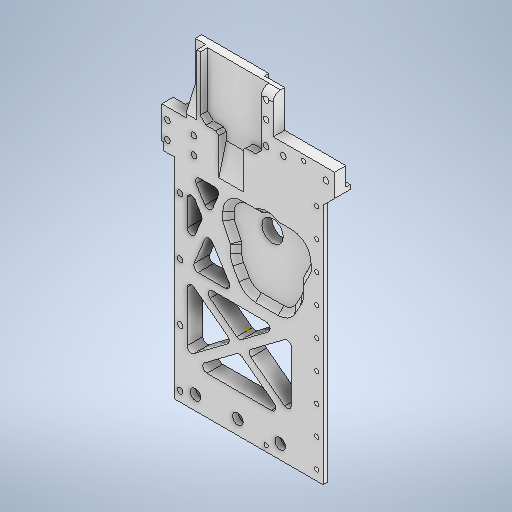
# Autodesk Inventor part: BottomSideMountRight
Saved by Autodesk Inventor 2026.2 (Build 302298000, 298)
## iProperties
Created: 2026-03-09
Part Number: BottomSideMountRight
Material: ABS Plastic
Document SubType Name: Modeling
Designer: gaoet
Density: 1.06 g/cm^3
Appearance: Smooth - White
Author: gaoet
Autodesk Inventor part; units mm, degrees
(part 1 of 2)
ref_plane "YZ Plane" through (0, 0, 0) normal (1, 0, 0) x (0, 1, 0)
ref_plane "XZ Plane" through (0, 0, 0) normal (0, 1, 0) x (-1, 0, 0)
ref_plane "XY Plane" through (0, 0, 0) normal (0, 0, 1) x (1, 0, 0)
sketch "Sketch1" plane through (0, 0, 0) normal (0, 0, 1) x (1, 0, 0)
  line L0 (56.625, -110) -> (-56.625, -110)
  line L1 (-56.625, -110) -> (-56.625, 110)
  line L2 (-56.625, 110) -> (56.625, 110)
  line L3 (56.625, 110) -> (56.625, -110)
  line L4 (56.625, -110) -> (-56.625, 110) construction
  line L5 (-56.625, -110) -> (56.625, 110) construction
  line L6 (-56.625, 110) -> (-47.875, 110)
  line L7 (-47.875, 110) -> (-47.875, 82)
  line L8 (-47.875, 82) -> (-56.625, 82)
  line L9 (-56.625, 82) -> (-56.625, 110)
  line L10 (-47.875, 82) -> (-47.875, -110)
  point P0 (0, 0)
  point P1 (-56.625, 82)
  dimension "d0" = 113.25
  dimension "d1" = 220
  dimension "d4" = 8.75
  dimension "d5" = 28
  constraints: 22 end point, 4 parallel, 2 horizontal, 2 midpoint, 2 perpendicular, 1 point on line, 1 vertical
  measures "d0" distance of L1.end L2.end
  measures "d1" distance of L0.end L1.end
  measures "d4" distance of L7.end L8.end
  measures "d5" distance of L6.end L7.end
extrude "Extrusion1" add sketch "Sketch1" along normal blind 8 contours L0 L10 L7 L2 L3 | L8 L1 L2 L7
sketch "Sketch2" plane through (0, 0, 8) normal (0, 0, 1) x (1, 0, 0)
  line L0 (-52.625, 102) -> (-34.125, 102)
  line L1 (-34.125, 102) -> (-34.125, 90)
  line L2 (-34.125, 90) -> (-52.625, 90)
  line L3 (-52.625, 90) -> (-52.625, 102)
  line L4 (-56.625, 110) -> (-56.625, 82) projected
  line L5 (56.625, 110) -> (-56.625, 110) projected
  point P0 (0, 0)
  dimension "d6" = 12
  dimension "d7" = 18.5
  dimension "d8" = 4
  dimension "d9" = 8
  constraints: 8 end point, 2 parallel, 1 horizontal, 1 perpendicular
  measures "d6" distance of L0.end L1.end
  measures "d7" distance of L0.start L0.end
  measures "d8" distance between parallel lines of L4 L3
  measures "d9" distance between parallel lines of L5 L0
hole "Hole1" at (-34.125, 102, 8) at (-34.125, 90, 8) at (-52.625, 90, 8) at (-52.625, 102, 8) direction (0, 0, -1) diameter 4 end through all
sketch "Sketch3" plane through (0, 0, 8) normal (0, 0, 1) x (1, 0, 0)
  circle A0 centre (-52.625, 102) radius 2 projected
  circle A1 centre (-52.625, 90) radius 2 projected
  circle A2 centre (-34.125, 90) radius 2 projected
  circle A3 centre (-34.125, 102) radius 2 projected
  line L0 (56.625, 110) -> (-56.625, 110) projected
  line L1 (-56.625, 110) -> (-56.625, 82) projected
  line L2 (-56.625, 82) -> (-47.875, 82) projected
  line L3 (-47.875, 82) -> (-47.875, -110) projected
  line L4 (-47.875, -110) -> (56.625, -110) projected
  line L5 (56.625, -110) -> (56.625, 110) projected
  line L6 (-56.625, 87.5) -> (-55.375, 87.5)
  line L7 (-55.375, 87.5) -> (-55.375, 82)
  point P0 (0, 0)
  dimension "d17" = 1.25
  dimension "d18" = 5.5
  constraints: 4 end point, 2 point on line, 1 horizontal, 1 perpendicular
  measures "d17" distance of L6.start L6.end
  measures "d18" distance of L6.end L7.end
extrude "Extrusion2" cut sketch "Sketch3" against normal blind 8 contours L6 L7 L2 L1
sketch "Sketch4" plane through (-47.875, -110, 0) normal (0, -1, 0) x (1, 0, 0)
  line L0 (0, 0) -> (104.5, 0) projected
  line L1 (104.5, 0) -> (104.5, 8) projected
  line L2 (0, 8) -> (104.5, 8) projected
  line L3 (0, 0) -> (0, 8) projected
  line L4 (104.5, 0) -> (89.25, 0)
  line L5 (89.25, 0) -> (89.25, 5)
  line L6 (89.25, 5) -> (104.5, 5)
  line L7 (104.5, 5) -> (104.5, 0)
  line L8 (89.25, 3.5) -> (95.5, 3.5)
  line L9 (95.5, 3.5) -> (95.5, 5)
  point P0 (47.875, 0)
  point P1 (89.25, 0)
  dimension "d21" = 15.25
  dimension "d22" = 5
  dimension "d25" = 1.5
  dimension "d26" = 9
  constraints: 12 end point, 2 horizontal, 2 parallel, 2 perpendicular, 2 point on line
  measures "d21" distance of L5.end L6.end
  measures "d22" distance of L4.end L5.end
  measures "d25" distance of L8.end L9.end
  measures "d26" distance between parallel lines of L1 L9
extrude "Extrusion3" cut sketch "Sketch4" against normal through all contours L5 L8 L9 L6 L1 L0
chamfer "Chamfer2" distance 5 angle 45 1 edges at (-51.625, 82, 0)
sketch "Sketch5" plane through (0, 0, 8) normal (0, 0, 1) x (1, 0, 0)
  line L0 (-56.625, 87.5) -> (-55.375, 87.5) projected
  line L1 (-55.375, 87.5) -> (-55.375, 82) projected
  line L2 (-55.375, 82) -> (-47.875, 82) projected
  line L3 (-47.875, 82) -> (-47.875, -110) projected
  line L4 (-47.875, -110) -> (56.625, -110) projected
  line L5 (56.625, -110) -> (56.625, 110) projected
  line L6 (56.625, 110) -> (-56.625, 110) projected
  line L7 (-56.625, 110) -> (-56.625, 87.5) projected
  circle A0 centre (-34.125, 102) radius 2 projected
  circle A1 centre (-34.125, 90) radius 2 projected
  circle A2 centre (-52.625, 90) radius 2 projected
  circle A3 centre (-52.625, 102) radius 2 projected
  line L8 (56.625, -65) -> (-47.875, -65)
  point P0 (0, 0)
  dimension "d33" = 45
  constraints: 2 end point, 2 point on line, 1 perpendicular
  measures "d33" distance between parallel lines of L8 L4
extrude "Extrusion4" cut sketch "Sketch5" against normal blind 25.4 contours L5 L4 L3 L8
sketch "Sketch6" plane through (-56.625, 110, 8) normal (0, 1, 0) x (1, 0, 0)
  line L0 (98, 4.5) -> (98, 8) projected
  line L1 (98, 8) -> (0, 8) projected
  line L2 (0, 8) -> (0, 0) projected
  line L3 (113.25, 0) -> (0, 0) projected
  line L4 (113.25, 3) -> (113.25, 0) projected
  line L5 (113.25, 3) -> (104.25, 3) projected
  line L6 (104.25, 3) -> (104.25, 4.5) projected
  line L7 (104.25, 4.5) -> (98, 4.5) projected
  line L8 (17, 0) -> (17, 8)
  line L9 (113.25, 3) -> (113.25, 8)
  line L10 (113.25, 8) -> (98, 8)
  point P0 (56.625, 8)
  point P1 (113.25, 1.5)
  dimension "d36" = 96.25
  constraints: 6 end point, 2 point on line, 1 horizontal, 1 midpoint, 1 perpendicular, 1 vertical
  measures "d36" distance from line of point (113.25, 1.5) L8
extrude "Extrusion5" add sketch "Sketch6" along normal blind 45 contours L7 L6 L5 L4 L3 L8 L1 L0 | L0 L10 L9 L5 L6 L7
sketch "Sketch7" plane through (0, 0, 8) normal (0, 0, 1) x (1, 0, 0)
  circle A0 centre (-52.625, 102) radius 2 projected
  circle A1 centre (-52.625, 90) radius 2 projected
  circle A2 centre (-34.125, 90) radius 2 projected
  circle A3 centre (-34.125, 102) radius 2 projected
  line L0 (-47.875, -65) -> (56.625, -65) projected
  line L1 (56.625, -65) -> (56.625, 155) projected
  line L2 (-39.625, 155) -> (56.625, 155) projected
  line L3 (-39.625, 110) -> (-39.625, 155) projected
  line L4 (-39.625, 110) -> (-56.625, 110) projected
  line L5 (-56.625, 110) -> (-56.625, 87.5) projected
  line L6 (-56.625, 87.5) -> (-55.375, 87.5) projected
  line L7 (-55.375, 87.5) -> (-55.375, 82) projected
  line L8 (-55.375, 82) -> (-47.875, 82) projected
  line L9 (-47.875, 82) -> (-47.875, -65) projected
  line L10 (56.625, 129) -> (21.625, 129)
  line L11 (21.625, 129) -> (21.625, 155)
  point P0 (0, 0)
  dimension "d39" = 26
  dimension "d40" = 35
  constraints: 4 end point, 2 point on line, 1 horizontal, 1 perpendicular
  measures "d39" distance of L10.end L11.end
  measures "d40" distance of L10.start L10.end
extrude "Extrusion6" cut sketch "Sketch7" against normal blind 25.4 contours L10 L11 L2 L1
sketch "Sketch8" plane through (0, 0, 8) normal (0, 0, 1) x (1, 0, 0)
  line L0 (56.625, 129) -> (21.625, 129) projected
  line L1 (21.625, 129) -> (21.625, 155) projected
  line L2 (56.625, -65) -> (56.625, 129) projected
  line L3 (-39.625, 155) -> (21.625, 155) projected
  point P0 (0, 0)
  point P1 (28.625, 121)
  point P2 (16.625, 121)
  point P3 (16.625, 137)
  point P4 (16.625, 149)
  point P5 (50.625, 121)
  point P6 (50.625, 121)
  dimension "d46" = 8
  dimension "d47" = 5
  dimension "d49" = 6
  dimension "d50" = 12
  dimension "d51" = 12
  dimension "d59" = 0
  dimension "d60" = 16
  dimension "d94" = 34
  constraints: 2 horizontal alignment, 2 vertical alignment, 1 coincident
  measures "d46" distance from line of L0 point (16.625, 121)
  measures "d47" distance from line of L1 point (16.625, 137)
  measures "d49" distance from line of L3 point (16.625, 149)
  measures "d50" distance of point (16.625, 149) point (16.625, 137)
  measures "d51" distance of point (28.625, 121) point (16.625, 121)
  measures "d59" horizontal distance of point (16.625, 137) point (16.625, 121)
  measures "d60" distance of point (16.625, 137) point (16.625, 121)
  measures "d94" distance of point (16.625, 121) point (50.625, 121)
hole "Hole2" at (28.625, 121, 8) at (16.625, 121, 8) at (16.625, 137, 8) at (16.625, 149, 8) direction (0, 0, -1) diameter 4 end through all
sketch "Sketch11" plane through (56.625, 110, 5) normal (1, 0, 0) x (0, 0, -1)
  line L0 (5, 19) -> (-3, 19) projected
  line L1 (-3, -175) -> (-3, 19) projected
  line L2 (-3, -175) -> (0, -175) projected
  line L3 (0, -175) -> (0, 0) projected
  line L4 (0, 0) -> (5, 0) projected
  line L5 (5, 0) -> (5, 19) projected
  line L6 (0, -175) -> (0, 0) projected
  line L7 (0, -30) -> (5, -30)
  line L8 (1.5, -175) -> (5, -175) projected
  line L9 (5, 0) -> (5, -175) projected
  line L10 (1.5, 0) -> (5, 0) projected
  line L11 (1.5, -175) -> (1.5, 0) projected
  point P0 (5, -110)
  point P1 (0, -30)
  dimension "d71" = 30
  constraints: 2 end point, 1 horizontal, 1 point on line
  measures "d71" distance between parallel lines of L4 L7
extrude "Extrusion9" add sketch "Sketch11" against normal up to surface (15.25 mm away) contours L9 L7 L11 L4 | L11 L7 L3 L4
sketch "Sketch13" plane through (-47.875, -65, 8) normal (0, -1, 0) x (1, 0, 0)
  line L0 (89.25, -8) -> (0, -8) projected
  line L1 (89.25, -4.5) -> (89.25, -8) projected
  line L2 (95.5, -4.5) -> (89.25, -4.5) projected
  line L3 (95.5, -3) -> (95.5, -4.5) projected
  line L4 (104.5, -3) -> (95.5, -3) projected
  line L5 (104.5, 0) -> (104.5, -3) projected
  line L6 (0, 0) -> (104.5, 0) projected
  line L7 (0, -8) -> (0, 0) projected
  line L8 (95.5, -4.5) -> (95.5, -7.5)
  line L9 (95.5, -7.5) -> (104.5, -7.5)
  line L10 (95.5, -7.5) -> (95.5, -8)
  line L11 (95.5, -4.5) -> (95.5, -3) projected
  line L12 (89.25, -4.5) -> (95.5, -4.5) projected
  line L13 (89.25, -8) -> (89.25, -4.5) projected
  line L14 (104.5, -8) -> (89.25, -8) projected
  line L15 (104.5, -3) -> (104.5, -8) projected
  line L16 (95.5, -3) -> (104.5, -3) projected
  point P0 (47.875, -8)
  dimension "d77" = 4.5
  constraints: 6 end point, 2 perpendicular, 2 point on line, 2 vertical
  measures "d77" distance between parallel lines of L4 L9
extrude "Extrusion11" [suppressed]
sketch "Sketch14" plane through (0, 0, 0) normal (0, 0, -1) x (-1, 0, 0)
  line L0 (-56.625, 80) -> (-56.625, 129) projected
  line L1 (-21.625, 129) -> (-56.625, 129) projected
  point P0 (0, 0)
  point P1 (-53.125, 125)
  point P2 (-42.875, 125)
  dimension "d81" = 3.5
  dimension "d82" = 4
  dimension "d83" = 10.25
  constraints: 1 horizontal alignment
  measures "d81" distance from line of L0 point (-53.125, 125)
  measures "d82" distance from line of L1 point (-53.125, 125)
  measures "d83" distance of point (-42.875, 125) point (-53.125, 125)
hole "Hole3" at (42.875, 125, 0) direction (0, 0, 1) diameter 3 end through all
sketch "Sketch15" plane through (0, 0, 0) normal (0, 0, -1) x (-1, 0, 0)
  circle A0 centre (-42.875, 125) radius 1.5 projected
  circle A1 centre (-16.625, 149) radius 2 projected
  circle A2 centre (-16.625, 137) radius 2 projected
  circle A3 centre (-16.625, 121) radius 2 projected
  circle A4 centre (-28.625, 121) radius 2 projected
  line L0 (-21.625, 155) -> (-21.625, 129) projected
  line L1 (-21.625, 129) -> (-56.625, 129) projected
  line L2 (-56.625, 80) -> (-56.625, 129) projected
  line L3 (-56.625, 80) -> (-41.375, 80) projected
  line L4 (-41.375, -65) -> (47.875, -65) projected
  line L5 (47.875, 87) -> (47.875, -65) projected
  line L6 (55.375, 87) -> (47.875, 87) projected
  line L7 (55.375, 87) -> (55.375, 87.5) projected
  line L8 (55.375, 87.5) -> (56.625, 87.5) projected
  line L9 (56.625, 110) -> (56.625, 87.5) projected
  line L10 (39.625, 110) -> (56.625, 110) projected
  line L11 (39.625, 110) -> (39.625, 155) projected
  line L12 (-21.625, 155) -> (39.625, 155) projected
  circle A5 centre (52.625, 102) radius 2 projected
  circle A6 centre (52.625, 90) radius 2 projected
  circle A7 centre (34.125, 90) radius 2 projected
  circle A8 centre (34.125, 102) radius 2 projected
  line L13 (-51.5517, 125.725) -> (-49.9784, 123)
  line L14 (-49.9784, 123) -> (-51.5517, 120.275)
  line L15 (-51.5517, 120.275) -> (-54.6983, 120.275)
  line L16 (-54.6983, 120.275) -> (-56.2716, 123)
  line L17 (-56.2716, 123) -> (-54.6983, 125.725)
  line L18 (-54.6983, 125.725) -> (-51.5517, 125.725)
  line L19 (-41.3017, 127.725) -> (-39.7284, 125)
  line L20 (-39.7284, 125) -> (-41.3017, 122.275)
  line L21 (-41.3017, 122.275) -> (-44.4483, 122.275)
  line L22 (-44.4483, 122.275) -> (-46.0216, 125)
  line L23 (-46.0216, 125) -> (-44.4483, 127.725)
  line L24 (-44.4483, 127.725) -> (-41.3017, 127.725)
  line L25 (-41.375, 80) -> (-41.375, -65) projected
  point P0 (0, 0)
  point P1 (-53.125, 123)
  dimension "d91" = 5.45
  constraints: 24 end point, 2 horizontal, 1 coincident, 1 equal length, 26 other
  measures "d91" distance between parallel lines of L15 L18
extrude "Extrusion12" cut sketch "Sketch15" against normal blind 2.5 contours A0 | L19 L20 L21 L22 L23 L24
sketch "Sketch16" plane through (0, 0, 8) normal (0, 0, 1) x (1, 0, 0)
  circle A0 centre (42.875, 125) radius 1.5 projected
  circle A1 centre (16.625, 149) radius 2 projected
  circle A2 centre (16.625, 137) radius 2 projected
  circle A3 centre (16.625, 121) radius 2 projected
  circle A4 centre (28.625, 121) radius 2 projected
  line L0 (56.625, 129) -> (21.625, 129) projected
  line L1 (21.625, 129) -> (21.625, 155) projected
  line L2 (-39.625, 155) -> (21.625, 155) projected
  line L3 (-39.625, 110) -> (-39.625, 155) projected
  line L4 (-39.625, 110) -> (-56.625, 110) projected
  line L5 (-56.625, 110) -> (-56.625, 87.5) projected
  line L6 (-56.625, 87.5) -> (-55.375, 87.5) projected
  line L7 (-55.375, 87.5) -> (-55.375, 82) projected
  line L8 (-55.375, 82) -> (-47.875, 82) projected
  line L9 (-47.875, 82) -> (-47.875, -65) projected
  line L10 (-47.875, -65) -> (56.625, -65) projected
  line L11 (56.625, -65) -> (56.625, 129) projected
  circle A5 centre (-34.125, 102) radius 2 projected
  circle A6 centre (-34.125, 90) radius 2 projected
  circle A7 centre (-52.625, 90) radius 2 projected
  circle A8 centre (-52.625, 102) radius 2 projected
  line L12 (56.625, 129) -> (64.625, 129)
  line L13 (64.625, 129) -> (64.625, 113)
  line L14 (64.625, 113) -> (56.625, 113)
  circle A9 centre (58.625, 121) radius 2
  point P0 (0, 0)
  point P1 (56.625, 121)
  dimension "d98" = 8
  dimension "d104" = 8
  dimension "d105" = 8
  dimension "d106" = 2
  constraints: 6 end point, 2 perpendicular, 1 centre point, 1 coincident, 1 equal radius, 1 horizontal, 1 point on line
  measures "d98" distance of L0.start L12.end
  measures "d104" distance from line of L0 A9.centre
  measures "d105" distance from line of A9.centre L14
  measures "d106" distance from line of L11 A9.centre
extrude "Extrusion13" add sketch "Sketch16" against normal up to surface (8 mm away) contours L12 L13 L14 L11
chamfer "Chamfer4" distance 8 angle 45 1 edges at (56.625, 113, 4)
sketch "Sketch17" plane through (56.625, 80, 0) normal (0, -1, 0) x (1, 0, 0)
  line L0 (-9, 3.5) -> (-9, 5) projected
  line L1 (-15.25, 3.5) -> (-9, 3.5) projected
  line L2 (-15.25, 0) -> (-15.25, 3.5) projected
  line L3 (0, 0) -> (-15.25, 0) projected
  line L4 (0, 5) -> (0, 0) projected
  line L5 (-9, 5) -> (0, 5) projected
  point P0 (-56.625, 0)
extrude "Extrusion14" cut sketch "Sketch17" against normal blind 27
sketch "Sketch18" plane through (0, 0, 8) normal (0, 0, 1) x (1, 0, 0)
  circle A0 centre (17.125, 67.6) radius 7.5
  line L0 (56.625, -65) -> (56.625, 105) projected
  line L1 (-39.625, 155) -> (21.625, 155) projected
  line L2 (-7.375, 72.6) -> (41.625, 72.6)
  line L3 (41.625, 72.6) -> (41.625, 28.6)
  line L4 (41.625, 28.6) -> (-7.375, 28.6)
  line L5 (-7.375, 28.6) -> (-7.375, 72.6)
  line L6 (-7.375, 61.6) -> (8.125, 28.6)
  line L7 (41.625, 61.6) -> (26.125, 28.6)
  line L8 (-1.9735, 50.1) -> (36.2235, 50.1)
  line L9 (-1.9735, 50.1) -> (-1.9735, 41.1)
  line L10 (-1.9735, 41.1) -> (5.125, 28.6)
  line L11 (36.2235, 50.1) -> (36.2235, 41.1)
  line L12 (36.2235, 41.1) -> (29.125, 28.6)
  point P0 (0, 0)
  point P1 (-9, 155)
  dimension "d109" = 39.5
  dimension "d110" = 87.4
  dimension "d111" = 15
  dimension "d112" = 49
  dimension "d113" = 39
  dimension "d114" = 24.5
  dimension "d115" = 11
  dimension "d116" = 18
  dimension "d119" = 5
  dimension "d120" = 17.5
  dimension "d121" = 9
  dimension "d122" = 24
  constraints: 22 end point, 8 point on line, 2 equal length, 2 horizontal, 2 horizontal alignment, 2 parallel, 2 vertical, 1 centre point, 1 midpoint, 1 perpendicular
  measures "d109" distance from line of A0.centre L0
  measures "d110" vertical distance of point (-9, 155) A0.centre
  measures "d111" diameter of A0
  measures "d112" distance of L3.end L4.end
  measures "d113" distance from line of L4 A0.centre
  measures "d114" distance from line of L3 A0.centre
  measures "d115" distance of L2.start L6.start
  measures "d116" distance of L7.end L6.end
  measures "d119" distance from line of A0.centre L2
  measures "d120" distance from line of A0.centre L8
  measures "d121" distance of L8.start L9.end
  measures "d122" distance of L12.end L10.end
extrude "Extrusion15" cut sketch "Sketch18" against normal blind 4 contours A0 L2 | A0 L2 L3 L7 L8 L6 L5 | L11 L12 L4 L7 | L7 L4 L6 L8 | L6 L4 L10 L9 picked at (19.5586, 67.0082)
fillet "Fillet1" radius 7 2 edges at (41.625, 72.6, 6) (-7.375, 72.6, 6)
extrude "Extrusion16" cut sketch "Sketch18" against normal blind 17.5 contours A0 L2 | L2 A0
fillet "Fillet2" radius 7 8 edges at (-1.9735, 50.1, 6) (-1.9735, 41.1, 6) (36.2235, 50.1, 6) (36.2235, 41.1, 6) (5.125, 28.6, 6) (29.125, 28.6, 6) (11.5348, 72.6, 6) (22.7152, 72.6, 6)
sketch "Sketch20" plane through (0, 0, 0) normal (0, 0, -1) x (-1, 0, 0)
  line L0 (47.875, 87) -> (47.875, -65) projected
  line L1 (-41.375, -65) -> (47.875, -65) projected
  point P0 (0, 0)
  point P1 (43.75, 62)
  point P2 (43.75, 22)
  point P3 (43.75, -18)
  point P4 (43.75, -58)
  dimension "d129" = 40
  dimension "d130" = 40
  dimension "d131" = 40
  dimension "d132" = 4.125
  dimension "d133" = 7
  constraints: 3 vertical alignment
  measures "d129" distance of point (43.75, 22) point (43.75, 62)
  measures "d130" distance of point (43.75, 22) point (43.75, -18)
  measures "d131" distance of point (43.75, -58) point (43.75, -18)
  measures "d132" distance from line of L0 point (43.75, 22)
  measures "d133" distance from line of L1 point (43.75, -58)
hole "Hole4" at (-43.75, 62, 0) at (-43.75, 22, 0) at (-43.75, -18, 0) at (-43.75, -58, 0) direction (0, 0, 1) diameter 4 depth 12
sketch "Sketch21" plane through (56.625, -65, 5) normal (0, 0, -1) x (-1, 0, 0)
  point P0 (56.625, 65)
sketch "Sketch22" plane through (56.625, -65, 5) normal (0, 0, -1) x (-1, 0, 0)
  line L0 (0, 170) -> (0, 172) projected
  line L1 (0, 0) -> (9, 0) projected
  line L2 (9, 0) -> (9, 172) projected
  line L3 (9, 172) -> (0, 172) projected
  line L4 (0, 0) -> (0, 170) projected
  point P0 (56.625, 65)
  point P1 (4.5, 167)
  point P2 (4.5, 147)
  point P3 (4.5, 127)
  point P4 (4.5, 107)
  point P5 (4.5, 87)
  point P6 (4.5, 67)
  point P7 (4.5, 47)
  point P8 (4.5, 27)
  point P9 (4.5, 7)
  point P10 (4.5, -13)
  point P11 (4.5, -33)
  dimension "d141" = 5
  dimension "d142" = 9
  dimension "d143" = 4.5
  dimension "d146" = 20
  constraints: 1 vertical, 10 other
  measures "d141" distance from line of L3 point (4.5, 167)
  measures "d142" distance of L2.end L0.end
  measures "d143" distance from line of point (4.5, 167) L2
  measures "d146" distance of point (4.5, 167) point (4.5, 147)
hole "Hole5" at (52.125, -98, 5) at (52.125, -58, 5) at (52.125, -38, 5) at (52.125, -18, 5) at (52.125, 2, 5) at (52.125, 22, 5) at (52.125, 42, 5) at (52.125, 62, 5) at (52.125, 82, 5) at (52.125, 102, 5) direction (0, 0, 1) diameter 3 depth 12
sketch "Sketch23" plane through (0, 0, 0) normal (0, 0, -1) x (-1, 0, 0)
  circle A0 centre (43.75, -58) radius 2 projected
  circle A1 centre (43.75, -18) radius 2 projected
  circle A2 centre (43.75, 22) radius 2 projected
  circle A3 centre (43.75, 62) radius 2 projected
  circle A4 centre (-17.125, 67.6) radius 7.5 projected
  circle A5 centre (34.125, 102) radius 2 projected
  circle A6 centre (34.125, 90) radius 2 projected
  circle A7 centre (52.625, 90) radius 2 projected
  circle A8 centre (52.625, 102) radius 2 projected
  circle A9 centre (-58.625, 121) radius 2 projected
  circle A10 centre (-28.625, 121) radius 2 projected
  circle A11 centre (-16.625, 121) radius 2 projected
  circle A12 centre (-16.625, 137) radius 2 projected
  circle A13 centre (-16.625, 149) radius 2 projected
  line L0 (-44.4483, 122.275) -> (-46.0216, 125) projected
  line L1 (-46.0216, 125) -> (-44.4483, 127.725) projected
  line L2 (-44.4483, 127.725) -> (-41.3017, 127.725) projected
  line L3 (-41.3017, 127.725) -> (-39.7284, 125) projected
  line L4 (-39.7284, 125) -> (-41.3017, 122.275) projected
  line L5 (-41.3017, 122.275) -> (-44.4483, 122.275) projected
  line L6 (-56.625, 105) -> (-56.625, 107) projected
  line L7 (-56.625, 107) -> (-41.375, 107) projected
  line L8 (-41.375, 107) -> (-41.375, -65) projected
  line L9 (-41.375, -65) -> (47.875, -65) projected
  line L10 (47.875, 87) -> (47.875, -65) projected
  line L11 (55.375, 87) -> (47.875, 87) projected
  line L12 (55.375, 87) -> (55.375, 87.5) projected
  line L13 (55.375, 87.5) -> (56.625, 87.5) projected
  line L14 (56.625, 110) -> (56.625, 87.5) projected
  line L15 (39.625, 110) -> (56.625, 110) projected
  line L16 (39.625, 110) -> (39.625, 155) projected
  line L17 (-21.625, 155) -> (39.625, 155) projected
  line L18 (-21.625, 155) -> (-21.625, 129) projected
  line L19 (-21.625, 129) -> (-64.625, 129) projected
  line L20 (-64.625, 129) -> (-64.625, 113) projected
  line L21 (-56.625, 105) -> (-64.625, 113) projected
  line L22 (-64.625, 155) -> (-7.625, 155)
  line L23 (-7.625, 155) -> (-7.625, 116)
  line L24 (-7.625, 116) -> (-64.625, 116)
  line L25 (-64.625, 116) -> (-64.625, 155)
  line L26 (-21.625, 155) -> (39.625, 155) projected
  line L27 (47.875, 87) -> (47.875, 110)
  point P0 (0, 0)
  point P1 (-7.625, 155)
  dimension "d158" = 39
  dimension "d159" = 14
  constraints: 10 end point, 2 parallel, 1 collinear, 1 horizontal, 1 perpendicular, 1 point on line, 1 vertical, 1 vertical alignment
  measures "d158" distance of L22.end L23.end
  measures "d159" distance between parallel lines of L18 L23
extrude "Extrusion18" add sketch "Sketch23" along normal blind 3 contours L21 L20 L24 L23 L17 L16 L15 L27 L10 L9 L8 L7 L6
sketch "Sketch24" plane through (0, 0, -3) normal (0, 0, -1) x (-1, 0, 0)
  line L0 (-56.625, 105) -> (-56.625, 107) projected
  line L1 (-56.625, 107) -> (-41.375, 107) projected
  line L2 (-41.375, 107) -> (-41.375, -65) projected
  line L3 (-41.375, -65) -> (47.875, -65) projected
  line L4 (47.875, -65) -> (47.875, 110) projected
  line L5 (47.875, 110) -> (39.625, 110) projected
  line L6 (39.625, 110) -> (39.625, 155) projected
  line L7 (39.625, 155) -> (-7.625, 155) projected
  line L8 (-7.625, 155) -> (-7.625, 116) projected
  line L9 (-7.625, 116) -> (-64.625, 116) projected
  line L10 (-64.625, 116) -> (-64.625, 113) projected
  line L11 (-64.625, 113) -> (-56.625, 105) projected
  circle A0 centre (34.125, 90) radius 2 projected
  circle A1 centre (34.125, 102) radius 2 projected
  circle A2 centre (-17.125, 67.6) radius 7.5 projected
  circle A3 centre (43.75, 62) radius 2 projected
  circle A4 centre (43.75, 22) radius 2 projected
  circle A5 centre (43.75, -18) radius 2 projected
  circle A6 centre (43.75, -58) radius 2 projected
  line L12 (47.875, -45) -> (-41.375, -45)
  line L13 (39.625, -65) -> (39.625, -45)
  point P0 (0, 0)
  dimension "d162" = 20
  dimension "d177" = 4.125
  dimension "d178" = 4.125
  constraints: 4 end point, 4 point on line, 1 horizontal, 1 vertical
  measures "d162" distance between parallel lines of L3 L12
  measures "d177" distance from line of L4 A6.centre
  measures "d178" distance from line of L13 A6.centre
extrude "Extrusion19" cut sketch "Sketch24" against normal blind 5 contours L12 L13 L3 L2
sketch "Sketch25" plane through (0, 0, 2) normal (0, 0, -1) x (-1, 0, 0)
  line L0 (-41.375, -45) -> (39.625, -45) projected
  line L1 (-41.375, -65) -> (-41.375, -45) projected
  line L2 (39.625, -65) -> (-41.375, -65) projected
  line L3 (39.625, -45) -> (39.625, -65) projected
  point P0 (0, 0)
  point P1 (33, -55)
  point P2 (3.25, -55)
  point P3 (-26.5, -55)
  dimension "d165" = 10
  dimension "d168" = 29.75
  dimension "d169" = 29.75
  constraints: 2 horizontal alignment
  measures "d165" distance from line of L2 point (33, -55)
  measures "d168" distance of point (3.25, -55) point (33, -55)
  measures "d169" distance of point (-26.5, -55) point (3.25, -55)
hole "Hole6" at (-33, -55, 2) at (26.5, -55, 2) at (-3.25, -55, 2) direction (0, 0, 1) diameter 4 depth 30
chamfer "Chamfer5" distance 10 angle 45 1 edges at (-39.625, -45, -0.5)
sketch "Sketch26" plane through (0, 0, 8) normal (0, 0, 1) x (1, 0, 0)
  line L0 (-47.875, -65) -> (56.625, -65) projected
  line L1 (56.625, -65) -> (56.625, 105) projected
  point P0 (0, 0)
  point P1 (16.625, -61)
  dimension "d182" = 4
  dimension "d183" = 40
  measures "d182" distance from line of L0 point (16.625, -61)
  measures "d183" distance from line of L1 point (16.625, -61)
hole "Hole7" at (16.625, -61, 8) direction (0, 0, -1) diameter 3 end through all
sketch "Sketch28" plane through (0, 0, -3) normal (0, 0, -1) x (-1, 0, 0)
  line L0 (39.625, -55) -> (39.625, -65) projected
  line L1 (39.625, -65) -> (47.875, -65) projected
  line L2 (47.875, -65) -> (47.875, 110) projected
  line L3 (47.875, 110) -> (39.625, 110) projected
  line L4 (39.625, 110) -> (39.625, 155) projected
  line L5 (39.625, 155) -> (-7.625, 155) projected
  line L6 (-7.625, 155) -> (-7.625, 116) projected
  line L7 (-7.625, 116) -> (-64.625, 116) projected
  line L8 (-64.625, 116) -> (-64.625, 113) projected
  line L9 (-64.625, 113) -> (-56.625, 105) projected
  line L10 (-56.625, 105) -> (-56.625, 107) projected
  line L11 (-56.625, 107) -> (-41.375, 107) projected
  line L12 (-41.375, 107) -> (-41.375, -45) projected
  line L13 (-41.375, -45) -> (29.625, -45) projected
  line L14 (39.625, -55) -> (29.625, -45) projected
  circle A0 centre (34.125, 90) radius 2 projected
  circle A1 centre (34.125, 102) radius 2 projected
  circle A2 centre (-17.125, 67.6) radius 7.5 projected
  circle A3 centre (43.75, 62) radius 2 projected
  circle A4 centre (43.75, 22) radius 2 projected
  circle A5 centre (43.75, -18) radius 2 projected
  circle A6 centre (43.75, -58) radius 2 projected
  point P0 (0, 0)
hole "Hole8" at (-43.75, -58, -3) at (-43.75, -18, -3) at (-43.75, 22, -3) at (-43.75, 62, -3) direction (0, 0, 1) diameter 4 depth 12 counterbore diameter 7.25 counterbore depth 4
sketch "Sketch29" plane through (0, 0, 8) normal (0, 0, 1) x (1, 0, 0)
  circle A0 centre (16.625, -61) radius 1.5 projected
  circle A1 centre (-3.25, -55) radius 2 projected
  circle A2 centre (26.5, -55) radius 2 projected
  circle A3 centre (-33, -55) radius 2 projected
  circle A4 centre (52.125, 102) radius 1.5 projected
  circle A5 centre (52.125, 82) radius 1.5 projected
  circle A6 centre (52.125, 62) radius 1.5 projected
  circle A7 centre (52.125, 42) radius 1.5 projected
  circle A8 centre (52.125, 22) radius 1.5 projected
  circle A9 centre (52.125, 2) radius 1.5 projected
  circle A10 centre (52.125, -18) radius 1.5 projected
  circle A11 centre (52.125, -38) radius 1.5 projected
  circle A12 centre (52.125, -58) radius 1.5 projected
  circle A13 centre (-43.75, -58) radius 2 projected
  circle A14 centre (-43.75, -18) radius 2 projected
  circle A15 centre (-43.75, 22) radius 2 projected
  circle A16 centre (-43.75, 62) radius 2 projected
  arc A17 (21.335, 73.8069) -> (25.2644, 72.6) centre (25.2644, 79.6) ccw projected
  line L0 (25.2644, 72.6) -> (34.625, 72.6) projected
  arc A18 (41.625, 65.6) -> (34.625, 72.6) centre (34.625, 65.6) ccw projected
  line L1 (41.625, 65.6) -> (41.625, 61.6) projected
  line L2 (41.625, 61.6) -> (36.8876, 51.5139) projected
  arc A19 (36.8876, 51.5139) -> (36.2235, 48.5379) centre (43.2235, 48.5379) ccw projected
  line L3 (36.2235, 48.5379) -> (36.2235, 42.9489) projected
  arc A20 (35.3105, 39.4922) -> (36.2235, 42.9489) centre (29.2235, 42.9489) ccw projected
  line L4 (35.3105, 39.4922) -> (31.1372, 32.1433) projected
  arc A21 (25.0502, 28.6) -> (31.1372, 32.1433) centre (25.0502, 35.6) ccw projected
  line L5 (25.0502, 28.6) -> (9.1998, 28.6) projected
  arc A22 (3.1128, 32.1433) -> (9.1998, 28.6) centre (9.1998, 35.6) ccw projected
  line L6 (3.1128, 32.1433) -> (-1.0605, 39.4922) projected
  arc A23 (-1.9735, 42.9489) -> (-1.0605, 39.4922) centre (5.0265, 42.9489) ccw projected
  line L7 (-1.9735, 42.9489) -> (-1.9735, 48.5379) projected
  arc A24 (-1.9735, 48.5379) -> (-2.6376, 51.5139) centre (-8.9735, 48.5379) ccw projected
  line L8 (-2.6376, 51.5139) -> (-7.375, 61.6) projected
  line L9 (-7.375, 61.6) -> (-7.375, 65.6) projected
  arc A25 (-0.375, 72.6) -> (-7.375, 65.6) centre (-0.375, 65.6) ccw projected
  line L10 (-0.375, 72.6) -> (8.9856, 72.6) projected
  arc A26 (8.9856, 72.6) -> (12.915, 73.8069) centre (8.9856, 79.6) ccw projected
  arc A27 (21.335, 73.8069) -> (12.915, 73.8069) centre (17.125, 67.6) ccw projected
  circle A28 centre (58.625, 121) radius 2 projected
  circle A29 centre (42.875, 125) radius 1.5 projected
  circle A30 centre (16.625, 149) radius 2 projected
  circle A31 centre (16.625, 137) radius 2 projected
  circle A32 centre (16.625, 121) radius 2 projected
  circle A33 centre (28.625, 121) radius 2 projected
  line L11 (64.625, 113) -> (64.625, 129) projected
  line L12 (64.625, 129) -> (21.625, 129) projected
  line L13 (21.625, 129) -> (21.625, 155) projected
  line L14 (-39.625, 155) -> (21.625, 155) projected
  line L15 (-39.625, 110) -> (-39.625, 155) projected
  line L16 (-39.625, 110) -> (-56.625, 110) projected
  line L17 (-56.625, 110) -> (-56.625, 87.5) projected
  line L18 (-56.625, 87.5) -> (-55.375, 87.5) projected
  line L19 (-55.375, 87.5) -> (-55.375, 82) projected
  line L20 (-55.375, 82) -> (-47.875, 82) projected
  line L21 (-47.875, 82) -> (-47.875, -65) projected
  line L22 (-47.875, -65) -> (56.625, -65) projected
  line L23 (56.625, -65) -> (56.625, 105) projected
  line L24 (64.625, 113) -> (56.625, 105) projected
  circle A34 centre (-34.125, 102) radius 2 projected
  circle A35 centre (-34.125, 90) radius 2 projected
  circle A36 centre (-52.625, 90) radius 2 projected
  circle A37 centre (-52.625, 102) radius 2 projected
  line L25 (12.875, 155) -> (-29.125, 155)
  line L26 (-29.125, 155) -> (-29.125, 113)
  line L27 (-29.125, 113) -> (12.875, 113)
  line L28 (12.875, 113) -> (12.875, 155)
  line L29 (12.875, 155) -> (-29.125, 113) construction
  line L30 (-29.125, 155) -> (12.875, 113) construction
  line L31 (-39.625, 155) -> (21.625, 155) projected
  line L32 (13.375, 112.5) -> (-29.625, 112.5)
  line L33 (-29.625, 112.5) -> (-29.625, 155.5)
  line L34 (-29.625, 155.5) -> (13.375, 155.5)
  line L35 (13.375, 155.5) -> (13.375, 112.5)
  point P0 (0, 0)
  point P1 (-8.125, 134)
  point P2 (21.625, 142)
  point P3 (-29.625, 155)
  point P4 (13.375, 155)
  dimension "d199" = 42
  dimension "d200" = 42
  dimension "d201" = 8.75
  dimension "d204" = 0.5
  constraints: 20 end point, 4 parallel, 3 midpoint, 2 perpendicular, 1 collinear, 1 horizontal, 3 other
  measures "d199" distance of L27.end L26.end
  measures "d200" distance of L26.end L25.end
  measures "d201" distance from line of point (21.625, 142) L28
  measures "d204" distance between parallel lines of L27 L32
extrude "Extrusion20" cut sketch "Sketch29" against normal blind 5.2 contours L35 L32 L33 L14 L26 L27 L28 | L28 L27 L26 L14
chamfer "Chamfer6" distance 4 angle 45 2 edges at (-29.625, 112.5, 5.4) (13.375, 112.5, 5.4)
sketch "Sketch30" plane through (0, 0, 8) normal (0, 0, 1) x (1, 0, 0)
  circle A0 centre (-52.625, 102) radius 2 projected
  circle A1 centre (-52.625, 90) radius 2 projected
  circle A2 centre (-34.125, 90) radius 2 projected
  circle A3 centre (-34.125, 102) radius 2 projected
  line L0 (13.375, 155) -> (13.375, 116.5) projected
  line L1 (9.375, 112.5) -> (13.375, 116.5) projected
  line L2 (9.375, 112.5) -> (-25.625, 112.5) projected
  line L3 (-29.625, 116.5) -> (-25.625, 112.5) projected
  line L4 (-29.625, 116.5) -> (-29.625, 155) projected
  line L5 (-39.625, 155) -> (-29.625, 155) projected
  line L6 (-39.625, 110) -> (-39.625, 155) projected
  line L7 (-39.625, 110) -> (-56.625, 110) projected
  line L8 (-56.625, 110) -> (-56.625, 87.5) projected
  line L9 (-56.625, 87.5) -> (-55.375, 87.5) projected
  line L10 (-55.375, 87.5) -> (-55.375, 82) projected
  line L11 (-55.375, 82) -> (-47.875, 82) projected
  line L12 (-47.875, 82) -> (-47.875, -65) projected
  line L13 (-47.875, -65) -> (56.625, -65) projected
  line L14 (56.625, -65) -> (56.625, 105) projected
  line L15 (64.625, 113) -> (56.625, 105) projected
  line L16 (64.625, 113) -> (64.625, 129) projected
  line L17 (64.625, 129) -> (21.625, 129) projected
  line L18 (21.625, 129) -> (21.625, 155) projected
  line L19 (13.375, 155) -> (21.625, 155) projected
  circle A4 centre (28.625, 121) radius 2 projected
  circle A5 centre (16.625, 121) radius 2 projected
  circle A6 centre (16.625, 137) radius 2 projected
  circle A7 centre (16.625, 149) radius 2 projected
  circle A8 centre (42.875, 125) radius 1.5 projected
  circle A9 centre (58.625, 121) radius 2 projected
  arc A10 (21.335, 73.8069) -> (25.2644, 72.6) centre (25.2644, 79.6) ccw projected
  line L20 (25.2644, 72.6) -> (34.625, 72.6) projected
  arc A11 (41.625, 65.6) -> (34.625, 72.6) centre (34.625, 65.6) ccw projected
  line L21 (41.625, 65.6) -> (41.625, 61.6) projected
  line L22 (41.625, 61.6) -> (36.8876, 51.5139) projected
  arc A12 (36.8876, 51.5139) -> (36.2235, 48.5379) centre (43.2235, 48.5379) ccw projected
  line L23 (36.2235, 48.5379) -> (36.2235, 42.9489) projected
  arc A13 (35.3105, 39.4922) -> (36.2235, 42.9489) centre (29.2235, 42.9489) ccw projected
  line L24 (35.3105, 39.4922) -> (31.1372, 32.1433) projected
  arc A14 (25.0502, 28.6) -> (31.1372, 32.1433) centre (25.0502, 35.6) ccw projected
  line L25 (25.0502, 28.6) -> (9.1998, 28.6) projected
  arc A15 (3.1128, 32.1433) -> (9.1998, 28.6) centre (9.1998, 35.6) ccw projected
  line L26 (3.1128, 32.1433) -> (-1.0605, 39.4922) projected
  arc A16 (-1.9735, 42.9489) -> (-1.0605, 39.4922) centre (5.0265, 42.9489) ccw projected
  line L27 (-1.9735, 42.9489) -> (-1.9735, 48.5379) projected
  arc A17 (-1.9735, 48.5379) -> (-2.6376, 51.5139) centre (-8.9735, 48.5379) ccw projected
  line L28 (-2.6376, 51.5139) -> (-7.375, 61.6) projected
  line L29 (-7.375, 61.6) -> (-7.375, 65.6) projected
  arc A18 (-0.375, 72.6) -> (-7.375, 65.6) centre (-0.375, 65.6) ccw projected
  line L30 (-0.375, 72.6) -> (8.9856, 72.6) projected
  arc A19 (8.9856, 72.6) -> (12.915, 73.8069) centre (8.9856, 79.6) ccw projected
  arc A20 (21.335, 73.8069) -> (12.915, 73.8069) centre (17.125, 67.6) ccw projected
  circle A21 centre (-43.75, 62) radius 2 projected
  circle A22 centre (-43.75, 22) radius 2 projected
  circle A23 centre (-43.75, -18) radius 2 projected
  circle A24 centre (-43.75, -58) radius 2 projected
  circle A25 centre (52.125, -58) radius 1.5 projected
  circle A26 centre (52.125, -38) radius 1.5 projected
  circle A27 centre (52.125, -18) radius 1.5 projected
  circle A28 centre (52.125, 2) radius 1.5 projected
  circle A29 centre (52.125, 22) radius 1.5 projected
  circle A30 centre (52.125, 42) radius 1.5 projected
  circle A31 centre (52.125, 62) radius 1.5 projected
  circle A32 centre (52.125, 82) radius 1.5 projected
  circle A33 centre (52.125, 102) radius 1.5 projected
  circle A34 centre (-33, -55) radius 2 projected
  circle A35 centre (26.5, -55) radius 2 projected
  circle A36 centre (-3.25, -55) radius 2 projected
  circle A37 centre (16.625, -61) radius 1.5 projected
  line L31 (8.9856, 75.1) -> (-0.375, 75.1)
  arc A38 (-0.375, 75.1) -> (-9.875, 65.6) centre (-0.375, 65.6) ccw
  line L32 (-9.875, 65.6) -> (-9.875, 61.0421)
  line L33 (-9.875, 61.0421) -> (-4.9004, 50.451)
  arc A39 (-4.4735, 48.5379) -> (-4.9004, 50.451) centre (-8.9735, 48.5379) ccw
  line L34 (-4.4735, 48.5379) -> (-4.4735, 42.9489)
  arc A40 (-4.4735, 42.9489) -> (-3.2344, 38.2577) centre (5.0265, 42.9489) ccw
  line L35 (-3.2344, 38.2577) -> (0.9389, 30.9088)
  arc A41 (0.9389, 30.9088) -> (9.1998, 26.1) centre (9.1998, 35.6) ccw
  line L36 (9.1998, 26.1) -> (25.0502, 26.1)
  arc A42 (25.0502, 26.1) -> (33.3111, 30.9088) centre (25.0502, 35.6) ccw
  line L37 (33.3111, 30.9088) -> (37.4844, 38.2577)
  arc A43 (37.4844, 38.2577) -> (38.7235, 42.9489) centre (29.2235, 42.9489) ccw
  line L38 (38.7235, 42.9489) -> (38.7235, 48.5379)
  arc A44 (39.1504, 50.451) -> (38.7235, 48.5379) centre (43.2235, 48.5379) ccw
  line L39 (39.1504, 50.451) -> (44.125, 61.0421)
  line L40 (44.125, 61.0421) -> (44.125, 65.6)
  arc A45 (44.125, 65.6) -> (34.625, 75.1) centre (34.625, 65.6) ccw
  line L41 (34.625, 75.1) -> (25.2644, 75.1)
  arc A46 (22.7384, 75.8759) -> (25.2644, 75.1) centre (25.2644, 79.6) ccw
  arc A47 (22.7384, 75.8759) -> (11.5116, 75.8759) centre (17.125, 67.6) ccw
  arc A48 (8.9856, 75.1) -> (11.5116, 75.8759) centre (8.9856, 79.6) ccw
  point P0 (0, 0)
  dimension "d208" = 2.5
  constraints: 22 end point, 22 point on circle, 11 centre point, 21 other
  measures "d208" distance between parallel lines of L30 L31
extrude "Extrusion21" cut sketch "Sketch30" against normal up to surface (4 mm away) contours A48 A47 A46 L41 A45 L40 L39 A44 L38 A43 L37 A42 L36 A41 L35 A40 L34 A39 L33 L32 A38 L31
sketch "Sketch31" plane through (0, 0, 8) normal (0, 0, 1) x (1, 0, 0)
  line L0 (37.4844, 38.2577) -> (33.3111, 30.9088) projected
  arc A0 (25.0502, 26.1) -> (33.3111, 30.9088) centre (25.0502, 35.6) ccw projected
  line L1 (25.0502, 26.1) -> (9.1998, 26.1) projected
  arc A1 (0.9389, 30.9088) -> (9.1998, 26.1) centre (9.1998, 35.6) ccw projected
  line L2 (0.9389, 30.9088) -> (-3.2344, 38.2577) projected
  arc A2 (-4.4735, 42.9489) -> (-3.2344, 38.2577) centre (5.0265, 42.9489) ccw projected
  line L3 (-4.4735, 42.9489) -> (-4.4735, 48.5379) projected
  arc A3 (-4.4735, 48.5379) -> (-4.9004, 50.451) centre (-8.9735, 48.5379) ccw projected
  line L4 (-4.9004, 50.451) -> (-9.875, 61.0421) projected
  line L5 (-9.875, 61.0421) -> (-9.875, 65.6) projected
  arc A4 (-0.375, 75.1) -> (-9.875, 65.6) centre (-0.375, 65.6) ccw projected
  line L6 (-0.375, 75.1) -> (8.9856, 75.1) projected
  arc A5 (8.9856, 75.1) -> (11.5116, 75.8759) centre (8.9856, 79.6) ccw projected
  arc A6 (22.7384, 75.8759) -> (11.5116, 75.8759) centre (17.125, 67.6) ccw projected
  arc A7 (22.7384, 75.8759) -> (25.2644, 75.1) centre (25.2644, 79.6) ccw projected
  line L7 (25.2644, 75.1) -> (34.625, 75.1) projected
  arc A8 (44.125, 65.6) -> (34.625, 75.1) centre (34.625, 65.6) ccw projected
  line L8 (44.125, 65.6) -> (44.125, 61.0421) projected
  line L9 (44.125, 61.0421) -> (39.1504, 50.451) projected
  arc A9 (39.1504, 50.451) -> (38.7235, 48.5379) centre (43.2235, 48.5379) ccw projected
  line L10 (38.7235, 48.5379) -> (38.7235, 42.9489) projected
  arc A10 (37.4844, 38.2577) -> (38.7235, 42.9489) centre (29.2235, 42.9489) ccw projected
  circle A11 centre (-52.625, 102) radius 2 projected
  circle A12 centre (-52.625, 90) radius 2 projected
  circle A13 centre (-34.125, 90) radius 2 projected
  circle A14 centre (-34.125, 102) radius 2 projected
  line L11 (13.375, 155) -> (13.375, 116.5) projected
  line L12 (9.375, 112.5) -> (13.375, 116.5) projected
  line L13 (9.375, 112.5) -> (-25.625, 112.5) projected
  line L14 (-29.625, 116.5) -> (-25.625, 112.5) projected
  line L15 (-29.625, 116.5) -> (-29.625, 155) projected
  line L16 (-39.625, 155) -> (-29.625, 155) projected
  line L17 (-39.625, 110) -> (-39.625, 155) projected
  line L18 (-39.625, 110) -> (-56.625, 110) projected
  line L19 (-56.625, 110) -> (-56.625, 87.5) projected
  line L20 (-56.625, 87.5) -> (-55.375, 87.5) projected
  line L21 (-55.375, 87.5) -> (-55.375, 82) projected
  line L22 (-55.375, 82) -> (-47.875, 82) projected
  line L23 (-47.875, 82) -> (-47.875, -65) projected
  line L24 (-47.875, -65) -> (56.625, -65) projected
  line L25 (56.625, -65) -> (56.625, 105) projected
  line L26 (64.625, 113) -> (56.625, 105) projected
  line L27 (64.625, 113) -> (64.625, 129) projected
  line L28 (64.625, 129) -> (21.625, 129) projected
  line L29 (21.625, 129) -> (21.625, 155) projected
  line L30 (13.375, 155) -> (21.625, 155) projected
  circle A15 centre (28.625, 121) radius 2 projected
  circle A16 centre (16.625, 121) radius 2 projected
  circle A17 centre (16.625, 137) radius 2 projected
  circle A18 centre (16.625, 149) radius 2 projected
  circle A19 centre (42.875, 125) radius 1.5 projected
  circle A20 centre (58.625, 121) radius 2 projected
  circle A21 centre (-43.75, 62) radius 2 projected
  circle A22 centre (-43.75, 22) radius 2 projected
  circle A23 centre (-43.75, -18) radius 2 projected
  circle A24 centre (-43.75, -58) radius 2 projected
  circle A25 centre (52.125, -58) radius 1.5 projected
  circle A26 centre (52.125, -38) radius 1.5 projected
  circle A27 centre (52.125, -18) radius 1.5 projected
  circle A28 centre (52.125, 2) radius 1.5 projected
  circle A29 centre (52.125, 22) radius 1.5 projected
  circle A30 centre (52.125, 42) radius 1.5 projected
  circle A31 centre (52.125, 62) radius 1.5 projected
  circle A32 centre (52.125, 82) radius 1.5 projected
  circle A33 centre (52.125, 102) radius 1.5 projected
  circle A34 centre (-33, -55) radius 2 projected
  circle A35 centre (26.5, -55) radius 2 projected
  circle A36 centre (-3.25, -55) radius 2 projected
  circle A37 centre (16.625, -61) radius 1.5 projected
  line L31 (-16.625, 105) -> (0.375, 105)
  line L32 (0.375, 105) -> (0.375, 112.5)
  line L33 (0.375, 112.5) -> (-16.625, 112.5)
  line L34 (-16.625, 112.5) -> (-16.625, 105)
  line L35 (-16.625, 105) -> (0.375, 112.5) construction
  line L36 (0.375, 105) -> (-16.625, 112.5) construction
  point P0 (0, 0)
  point P1 (-8.125, 108.75)
  point P2 (-8.125, 112.5)
  dimension "d211" = 17
  dimension "d212" = 7.5
  constraints: 12 end point, 3 midpoint, 2 parallel, 1 horizontal, 1 perpendicular, 1 point on line, 1 vertical alignment
  measures "d211" distance of L31.start L31.end
  measures "d212" distance of L31.end L32.end
extrude "Extrusion22" cut sketch "Sketch31" against normal up to surface (5.2 mm away) contours L32 L31 L34 L13
chamfer "Chamfer7" distance 2 angle 45 2 edges at (-16.625, 112.5, 5.4) (0.375, 112.5, 5.4)
chamfer "Chamfer8" distance 20 distance2 5.2 1 edges at (-8.125, 105, 8) measured on face at (-8.125, 104.5, 8)
fillet "Fillet3" radius 5 1 edges at (17.5, 155, 8)
sketch "Sketch32" plane through (-56.625, 155, 8) normal (0, 1, 0) x (1, 0, 0)
  line L0 (17, 18.65) -> (-25.3, 18.65)
  line L1 (-25.3, 18.65) -> (-25.3, -23.65)
  line L2 (-25.3, -23.65) -> (17, -23.65)
  line L3 (17, -23.65) -> (17, 18.65)
  line L4 (17, 18.65) -> (-25.3, -23.65) construction
  line L5 (-25.3, 18.65) -> (17, -23.65) construction
  line L6 (17, 11) -> (64.25, 11) projected
  line L7 (78.25, 5) -> (70, 5) projected
  line L8 (78.25, 5) -> (78.25, 8) projected
  line L9 (78.25, 8) -> (64.25, 8) projected
  line L10 (64.25, 8) -> (64.25, 11) projected
  line L11 (17, 11) -> (64.25, 11) projected
  line L12 (17, 0) -> (17, 11) projected
  line L13 (17, 0) -> (27, 0) projected
  line L14 (27, 0) -> (27, 5.2) projected
  line L15 (27, 5.2) -> (70, 5.2) projected
  line L16 (70, 5.2) -> (70, 5) projected
  line L17 (23.5, 5.5) -> (17, 5.5)
  line L18 (17, 5.5) -> (17, -10.5)
  line L19 (17, -10.5) -> (23.5, -10.5)
  line L20 (23.5, -10.5) -> (23.5, 5.5)
  line L21 (23.5, 5.5) -> (17, -10.5) construction
  line L22 (17, 5.5) -> (23.5, -10.5) construction
  line L23 (24.5, 6.5) -> (16, 6.5)
  line L24 (16, 6.5) -> (16, -11.5)
  line L25 (16, -11.5) -> (24.5, -11.5)
  line L26 (24.5, -11.5) -> (24.5, 6.5)
  point P0 (56.625, 8)
  point P1 (-4.15, -2.5)
  point P2 (20.25, -2.5)
  dimension "d222" = 42.3
  dimension "d223" = 7.65
  dimension "d224" = 6.5
  dimension "d225" = 16
  dimension "d226" = 1
  constraints: 32 end point, 6 parallel, 4 midpoint, 4 perpendicular, 2 horizontal, 1 collinear, 1 horizontal alignment, 1 point on line, 3 other
  measures "d222" distance of L2.end L1.end
  measures "d223" distance between parallel lines of L6 L0
  measures "d224" distance of L19.end L18.end
  measures "d225" distance of L18.end L17.end
  measures "d226" distance between parallel lines of L20 L26
extrude "Extrusion23" cut sketch "Sketch32" against normal up to surface (42.5 mm away) contours L23 L26 L13 L20 L17 L3 | L3 L25 L24 L23 | L17 L20 L13 L3 | L3 L19 L20 L13 L26 L25 | L13 L20 L19 L3
chamfer "Chamfer9" distance 6.5 distance2 15 1 edges at (-35.875, 112.5, 1.5) measured on face at (-35.875, 112.5, 2)
sketch "Sketch33" plane through (0, 0, -3) normal (0, 0, -1) x (-1, 0, 0)
  circle A0 centre (43.75, 62) radius 3.625 projected
  circle A1 centre (43.75, 22) radius 3.625 projected
  circle A2 centre (43.75, -18) radius 3.625 projected
  circle A3 centre (43.75, -58) radius 3.625 projected
  line L0 (39.625, -55) -> (39.625, -65) projected
  line L1 (39.625, -65) -> (47.875, -65) projected
  line L2 (47.875, -65) -> (47.875, 110) projected
  line L3 (47.875, 110) -> (39.625, 110) projected
  line L4 (39.625, 110) -> (39.625, 155) projected
  line L5 (39.625, 155) -> (-7.625, 155) projected
  line L6 (-7.625, 155) -> (-7.625, 116) projected
  line L7 (-7.625, 116) -> (-64.625, 116) projected
  line L8 (-64.625, 116) -> (-64.625, 113) projected
  line L9 (-64.625, 113) -> (-56.625, 105) projected
  line L10 (-56.625, 105) -> (-56.625, 107) projected
  line L11 (-56.625, 107) -> (-41.375, 107) projected
  line L12 (-41.375, 107) -> (-41.375, -45) projected
  line L13 (-41.375, -45) -> (29.625, -45) projected
  line L14 (39.625, -55) -> (29.625, -45) projected
  circle A4 centre (34.125, 90) radius 2 projected
  circle A5 centre (34.125, 102) radius 2 projected
  circle A6 centre (-17.125, 67.6) radius 7.5 projected
  line L15 (-59.625, 108) -> (-47.625, 108)
  line L16 (-47.625, -65) -> (-47.625, 107) projected
  line L17 (-47.625, 108) -> (-47.625, 107)
  point P0 (0, 0)
  dimension "d232" = 1
  constraints: 4 end point, 1 horizontal, 1 point on line, 1 vertical
  measures "d232" distance between parallel lines of L11 L15
extrude "Extrusion24" cut sketch "Sketch33" against normal up to surface (8 mm away) contours L11 L10 L9 L15 L17
sketch "Sketch34" plane through (0, 0, 8) normal (0, 0, 1) x (1, 0, 0)
  line L0 (-32.125, 155) -> (-32.125, 112.5) projected
  line L1 (-32.125, 112.5) -> (-39.625, 112.5) projected
  line L2 (-39.625, 110) -> (-39.625, 112.5) projected
  line L3 (-39.625, 110) -> (-56.625, 110) projected
  line L4 (-56.625, 110) -> (-56.625, 87.5) projected
  line L5 (-56.625, 87.5) -> (-55.375, 87.5) projected
  line L6 (-55.375, 87.5) -> (-55.375, 82) projected
  line L7 (-55.375, 82) -> (-47.875, 82) projected
  line L8 (-47.875, 82) -> (-47.875, -65) projected
  line L9 (-47.875, -65) -> (56.625, -65) projected
  line L10 (56.625, -65) -> (56.625, 105) projected
  line L11 (64.625, 113) -> (56.625, 105) projected
  line L12 (64.625, 113) -> (64.625, 129) projected
  line L13 (64.625, 129) -> (21.625, 129) projected
  line L14 (21.625, 129) -> (21.625, 150) projected
  line L15 (18.3571, 150) -> (21.625, 150) projected
  arc A0 (14.8929, 150) -> (18.3571, 150) centre (16.625, 149) ccw projected
  line L16 (13.375, 150) -> (14.8929, 150) projected
  line L17 (13.375, 150) -> (13.375, 116.5) projected
  line L18 (9.375, 112.5) -> (13.375, 116.5) projected
  line L19 (9.375, 112.5) -> (2.375, 112.5) projected
  line L20 (0.375, 110.5) -> (2.375, 112.5) projected
  line L21 (0.375, 110.5) -> (0.375, 85) projected
  line L22 (-16.625, 85) -> (0.375, 85) projected
  line L23 (-16.625, 85) -> (-16.625, 110.5) projected
  line L24 (-18.625, 112.5) -> (-16.625, 110.5) projected
  line L25 (-18.625, 112.5) -> (-25.625, 112.5) projected
  line L26 (-29.625, 116.5) -> (-25.625, 112.5) projected
  line L27 (-29.625, 116.5) -> (-29.625, 155) projected
  line L28 (-32.125, 155) -> (-29.625, 155) projected
  circle A1 centre (16.625, -61) radius 1.5 projected
  circle A2 centre (-3.25, -55) radius 2 projected
  circle A3 centre (26.5, -55) radius 2 projected
  circle A4 centre (-33, -55) radius 2 projected
  circle A5 centre (52.125, 102) radius 1.5 projected
  circle A6 centre (52.125, 82) radius 1.5 projected
  circle A7 centre (52.125, 62) radius 1.5 projected
  circle A8 centre (52.125, 42) radius 1.5 projected
  circle A9 centre (52.125, 22) radius 1.5 projected
  circle A10 centre (52.125, 2) radius 1.5 projected
  circle A11 centre (52.125, -18) radius 1.5 projected
  circle A12 centre (52.125, -38) radius 1.5 projected
  circle A13 centre (52.125, -58) radius 1.5 projected
  circle A14 centre (-43.75, -58) radius 2 projected
  circle A15 centre (-43.75, -18) radius 2 projected
  circle A16 centre (-43.75, 22) radius 2 projected
  circle A17 centre (-43.75, 62) radius 2 projected
  circle A18 centre (58.625, 121) radius 2 projected
  circle A19 centre (42.875, 125) radius 1.5 projected
  circle A20 centre (16.625, 137) radius 2 projected
  circle A21 centre (16.625, 121) radius 2 projected
  circle A22 centre (28.625, 121) radius 2 projected
  circle A23 centre (-34.125, 102) radius 2 projected
  circle A24 centre (-34.125, 90) radius 2 projected
  circle A25 centre (-52.625, 90) radius 2 projected
  circle A26 centre (-52.625, 102) radius 2 projected
  line L29 (37.4844, 38.2577) -> (33.3111, 30.9088) projected
  arc A27 (25.0502, 26.1) -> (33.3111, 30.9088) centre (25.0502, 35.6) ccw projected
  line L30 (25.0502, 26.1) -> (9.1998, 26.1) projected
  arc A28 (0.9389, 30.9088) -> (9.1998, 26.1) centre (9.1998, 35.6) ccw projected
  line L31 (0.9389, 30.9088) -> (-3.2344, 38.2577) projected
  arc A29 (-4.4735, 42.9489) -> (-3.2344, 38.2577) centre (5.0265, 42.9489) ccw projected
  line L32 (-4.4735, 42.9489) -> (-4.4735, 48.5379) projected
  arc A30 (-4.4735, 48.5379) -> (-4.9004, 50.451) centre (-8.9735, 48.5379) ccw projected
  line L33 (-4.9004, 50.451) -> (-9.875, 61.0421) projected
  line L34 (-9.875, 61.0421) -> (-9.875, 65.6) projected
  arc A31 (-0.375, 75.1) -> (-9.875, 65.6) centre (-0.375, 65.6) ccw projected
  line L35 (-0.375, 75.1) -> (8.9856, 75.1) projected
  arc A32 (8.9856, 75.1) -> (11.5116, 75.8759) centre (8.9856, 79.6) ccw projected
  arc A33 (22.7384, 75.8759) -> (11.5116, 75.8759) centre (17.125, 67.6) ccw projected
  arc A34 (22.7384, 75.8759) -> (25.2644, 75.1) centre (25.2644, 79.6) ccw projected
  line L36 (25.2644, 75.1) -> (34.625, 75.1) projected
  arc A35 (44.125, 65.6) -> (34.625, 75.1) centre (34.625, 65.6) ccw projected
  line L37 (44.125, 65.6) -> (44.125, 61.0421) projected
  line L38 (44.125, 61.0421) -> (39.1504, 50.451) projected
  arc A36 (39.1504, 50.451) -> (38.7235, 48.5379) centre (43.2235, 48.5379) ccw projected
  line L39 (38.7235, 48.5379) -> (38.7235, 42.9489) projected
  arc A37 (37.4844, 38.2577) -> (38.7235, 42.9489) centre (29.2235, 42.9489) ccw projected
  point P0 (0, 0)
hole "Hole9" at (-3.25, -55, 8) at (26.5, -55, 8) at (-33, -55, 8) direction (0, 0, -1) diameter 3 end through all counterbore diameter 7.5 counterbore depth 4
chamfer "Chamfer10" distance 4 angle 45 22 edges at (23.9432, 75.2983, 8) (29.9447, 75.1, 8) (41.3425, 72.3175, 8) (44.125, 63.3211, 8) (17.125, 77.6, 8) (10.3068, 75.2983, 8) (4.3053, 75.1, 8) (-7.0925, 72.3175, 8) (-9.875, 63.3211, 8) (41.6377, 55.7466, 8) (38.8315, 49.518, 8) (38.7235, 45.7434, 8) (38.4085, 40.5229, 8) (35.3978, 34.5833, 8) (29.8295, 27.3898, 8) (17.125, 26.1, 8) (4.4205, 27.3898, 8) (-1.1478, 34.5833, 8) (-4.1585, 40.5229, 8) (-4.4735, 45.7434, 8) (-4.5815, 49.518, 8) (-7.3877, 55.7466, 8)